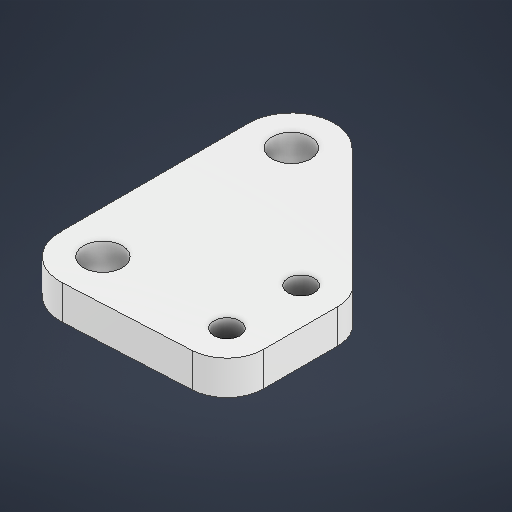
# Autodesk Inventor part: CNC-025-YAxisCableCarrierMount
Saved by Autodesk Inventor 2026.2 (Build 302298000, 298)
## iProperties
Created: 2026-06-25
Part Number: CNC-025-YAxisCableCarrierMount
Material: ABS Plastic
Document SubType Name: Modeling
Designer: Kenji
Density: 1.06 g/cm^3
Appearance: Smooth - White
Author: Kenji
Autodesk Inventor part; units mm, degrees
ref_plane "YZ Plane" through (0, 0, 0) normal (1, 0, 0) x (0, 1, 0)
ref_plane "XZ Plane" through (0, 0, 0) normal (0, 1, 0) x (-1, 0, 0)
ref_plane "XY Plane" through (0, 0, 0) normal (0, 0, 1) x (1, 0, 0)
sketch "Sketch1" plane through (0, 0, 0) normal (0, 1, 0) x (-1, 0, 0)
  circle A0 centre (0, 0) radius 2.6
  circle A1 centre (0, -25.4) radius 2.6
  circle A2 centre (-16.7115, 0) radius 1.75
  circle A3 centre (-16.7115, -10) radius 1.75
  circle A4 centre (0, 0) radius 5.775 construction
  circle A5 centre (0, -25.4) radius 5.775 construction
  circle A6 centre (-16.7115, 0) radius 4.925 construction
  circle A7 centre (-16.7115, -10) radius 4.925 construction
  line L0 (-0.2937, 5.7675) -> (-16.962, 4.9186)
  line L1 (5.775, 0) -> (5.775, -25.4)
  line L2 (-4.0696, -29.4974) -> (-20.1821, -13.4943)
  line L3 (-21.6365, 0) -> (-21.6365, -10)
  arc A8 (-4.0696, -29.4974) -> (5.775, -25.4) centre (0, -25.4) ccw
  arc A9 (5.775, 0) -> (-0.2937, 5.7675) centre (0, 0) ccw
  arc A10 (-16.962, 4.9186) -> (-21.6365, 0) centre (-16.7115, 0) ccw
  arc A11 (-21.6365, -10) -> (-20.1821, -13.4943) centre (-16.7115, -10) ccw
  dimension "d0" = 5.2
  dimension "d1" = 25.4
  dimension "d2" = 16.7115
  dimension "d3" = 3.5
  dimension "d4" = 10
  dimension "d5" = 3.175
  dimension "d6" = 3.175
  constraints: 16 point on circle, 12 centre point, 11 tangent, 8 end point, 7 equal radius, 2 coincident, 2 vertical alignment, 1 horizontal alignment, 1 vertical
  measures "d0" diameter of A0
  measures "d1" distance of A1.centre point (0, 0)
  measures "d2" distance of A2.centre point (0, 0)
  measures "d3" diameter of A2
  measures "d4" distance of A3.centre A2.centre
  measures "d5" radial gap between concentric circles of A0 A4
  measures "d6" radial gap between concentric circles of A6 A2
extrude "Extrusion1" add sketch "Sketch1" along normal blind 4.5994
equation "\"d6\" = d5"
body "Solid1"
